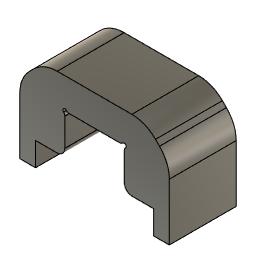
Y Linear Rail Jig v2 (Autodesk Fusion 360 design; units mm, degrees)
Autodesk Fusion 360 part; units mm, degrees
note: some values were not read from the file. Set by a fixed rule: which sketch regions a step uses.
sketch "Sketch1" plane through (0, 0, 0) normal (0, 1, 0) x (1, 0, 0)
  line L0 (0, 0) -> (4, 0)
  line L1 (4, 0) -> (4, -6)
  line L2 (4, -6) -> (11.45, -6)
  line L3 (11.45, -6) -> (11.45, -16.2)
  line L4 (11.45, -16.2) -> (26.55, -16.2)
  line L5 (26.55, -16.2) -> (26.55, -6)
  line L6 (26.55, -6) -> (34, -6)
  line L7 (34, -6) -> (34, 0)
  line L8 (34, 0) -> (38, 0)
  line L9 (38, 0) -> (38, -24)
  line L10 (38, -24) -> (0, -24)
  line L11 (0, -24) -> (0, 0)
  dimension "d1" = 15.1
  dimension "d2" = 10.2
  dimension "d3" = 30
  dimension "d4" = 6
  dimension "d5" = 4
  dimension "d6" = 24
  constraint coincident L0.start L11.end
  constraint horizontal L0
  constraint perpendicular L0 L1
  constraint perpendicular L1 L2
  constraint perpendicular L2 L3
  constraint perpendicular L3 L4
  constraint perpendicular L4 L5
  constraint perpendicular L5 L6
  constraint perpendicular L6 L7
  constraint perpendicular L5 L8
  constraint perpendicular L8 L9
  constraint perpendicular L9 L10
  constraint perpendicular L0 L11
  constraint equal L0 L8
  constraint equal L2 L6
  constraint equal L3 L5
  constraint equal L1 L7
  measures "d1" distance of L3.end L4.end
  measures "d2" distance of L2.end L3.end
  measures "d3" distance of L1 L7
  measures "d4" distance of L0.end L1.end
  measures "d5" distance of L0.start L0.end
  measures "d6" distance of L0 L10
extrude "Extrude1" add sketch "Sketch1" along normal blind 17
chamfer "Chamfer1" distance 6 distance2 6 2 edges at (38, 8.5, 24) (0, 8.5, 24) measured on face at (25.3333, 5.6667, 24) measured on face at (0, 5.6667, 16)
fillet "Fillet1" radius 2 2 edges at (11.45, 8.5, 6) (26.55, 8.5, 6)
sketch "Sketch2" plane through (0, 0, 0) normal (0, -1, 0) x (1, 0, 0)
  arc A0 (26.55, 8) -> (28.55, 6) centre (28.55, 8) ccw
  line L0 (28.55, 6) -> (34, 6)
  line L1 (34, 6) -> (34, 0)
  line L2 (34, 0) -> (38, 0)
  line L3 (38, 0) -> (38, 18)
  line L4 (38, 18) -> (32, 24)
  line L5 (32, 24) -> (6, 24)
  line L6 (6, 24) -> (0, 18)
  line L7 (0, 18) -> (0, 0)
  line L8 (0, 0) -> (4, 0)
  line L9 (4, 0) -> (4, 6)
  line L10 (4, 6) -> (9.45, 6)
  arc A1 (9.45, 6) -> (11.45, 8) centre (9.45, 8) ccw
  line L11 (11.45, 8) -> (11.45, 16.2)
  line L12 (11.45, 16.2) -> (26.55, 16.2)
  line L13 (26.55, 16.2) -> (26.55, 8)
  circle A2 centre (11.45, 16.2) radius 0.5
  circle A3 centre (26.55, 16.2) radius 0.5
  dimension "d13" = 1
  dimension "d14" = 1
  constraint coincident L11.end L12.start
  constraint coincident L12.end L13.start
  measures "d13" diameter of A2
  measures "d14" diameter of A3
extrude "Extrude2" cut sketch "Sketch2" against normal through all contours L12 L13 A3 | L11 L12 A2 picked at (26.2406, 16.3214) picked at (11.3772, 15.8756)
fillet "Fillet2" radius 1 4 edges at (11.45, 8.5, 15.7) (11.95, 8.5, 16.2) (26.05, 8.5, 16.2) (26.55, 8.5, 15.7)
fillet "Fillet5" radius 8.5 4 edges at (6, 8.5, 24) (0, 8.5, 18) (32, 8.5, 24) (38, 8.5, 18)
